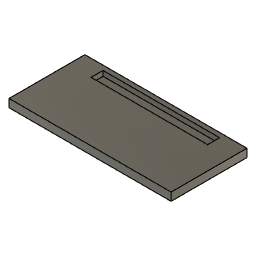
baseplate v3 (Autodesk Fusion 360 design; units mm, degrees)
Autodesk Fusion 360 part; units mm, degrees
sketch "Sketch1" plane through (0, 0, 0) normal (0, 0, 1) x (1, 0, 0)
  line L0 (0, 0) -> (70.5, 0)
  line L1 (70.5, 0) -> (70.5, 32)
  line L2 (70.5, 32) -> (0, 32)
  line L3 (0, 32) -> (0, 0)
  dimension "d1" = 70.5
  dimension "d2" = 32
  constraint horizontal L0
  constraint vertical L1
  constraint horizontal L2
  constraint vertical L3
  constraint coincident L0.start L3.end
  measures "d1" distance of L0.start L0.end
  measures "d2" distance of L0.start L2.end
extrude "Extrude1" add sketch "Sketch1" along normal blind 1.5
extrude "Extrude2" add 1 faces at (47, 32, 0.5) along direction (0, 1, 0) blind 1
extrude "Extrude3" add 1 faces at (23.5, 22, 1.5) along direction (0, 0, 1) blind 2
sketch "Sketch2" plane through (0, 0, 3.5) normal (0, 0, 1) x (-1, 0, 0)
  line L0 (0, -33) -> (0, 0)
  line L1 (0, 0) -> (-70.5, 0)
  line L2 (-70.5, 0) -> (-70.5, -33)
  line L3 (-70.5, -33) -> (0, -33)
  line L4 (-35.25, -33) -> (-35.25, -31)
  line L5 (-35.25, -31) -> (-35.25, -28.75)
  line L6 (-60.25, -26.5) -> (-10.25, -26.5)
  line L7 (-10.25, -26.5) -> (-10.25, -31)
  line L8 (-10.25, -31) -> (-60.25, -31)
  line L9 (-60.25, -31) -> (-60.25, -26.5)
  line L10 (-60.25, -26.5) -> (-10.25, -31) construction
  line L11 (-10.25, -26.5) -> (-60.25, -31) construction
  point P0 (-35.25, -28.75)
  dimension "d9" = 2
  dimension "d10" = 2.25
  dimension "d11" = 50
  dimension "d12" = 4.5
  constraint midpoint L3 L4.start
  constraint perpendicular L3 L4
  constraint perpendicular L3 L5
  constraint horizontal L6
  constraint perpendicular L6 L7
  constraint parallel L6 L8
  constraint parallel L7 L9
  constraint coincident L10 P0
  constraint coincident L11 P0
  constraint coincident P0 L5.end
  measures "d9" distance of L4.start L4.end
  measures "d10" distance of L4.end P0
  measures "d11" distance of L7.end L8.end
  measures "d12" distance of L6.end L7.end
extrude "Extrude4" cut sketch "Sketch2" against normal blind 2.2 contours L6 L7 L8 L9
extrude "Extrude5" cut 1 faces at (43.5833, 26.5, 2.7667) along direction (0, -1, 0) blind 0.7
extrude "Extrude6" cut 1 faces at (10.25, 27.5333, 2.7667) along direction (-1, 0, 0) blind 0.35
extrude "Extrude7" cut 1 faces at (60.25, 27.5333, 2.0333) along direction (1, 0, 0) blind 0.35
